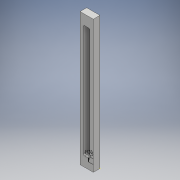
# Autodesk Inventor part: piças
Saved by Autodesk Inventor 2018 (Build 220112000, 112)
## iProperties
Created: 2018-03-15
Part Number: piças
Material: Genérico
Document SubType Name: Modeling
Designer: Georgines
Density: 1 g/cm^3
Appearance: Padrão
Author: Georgines
Autodesk Inventor part; units mm, degrees
ref_plane "YZ Plane" through (0, 0, 0) normal (1, 0, 0) x (0, 1, 0)
ref_plane "XZ Plane" through (0, 0, 0) normal (0, 1, 0) x (-1, 0, 0)
ref_plane "XY Plane" through (0, 0, 0) normal (0, 0, 1) x (1, 0, 0)
sketch "Esboço1" plane through (0, 0, 0) normal (0, 1, 0) x (-1, 0, 0)
  line L0 (-10, 100) -> (10, 100)
  line L1 (10, 100) -> (10, -100)
  line L2 (10, -100) -> (-10, -100)
  line L3 (-10, -100) -> (-10, 100)
  line L4 (-10, 100) -> (10, -100) construction
  line L5 (10, 100) -> (-10, -100) construction
  line L6 (-3, -85) -> (3, -85)
  line L7 (5, -83) -> (5, 83)
  line L8 (3, 85) -> (-3, 85)
  line L9 (-5, 83) -> (-5, -83)
  line L10 (-5, -85) -> (5, 85) construction
  line L11 (5, -85) -> (-5, 85) construction
  arc A0 (5, 83) -> (3, 85) centre (3, 83) ccw
  arc A1 (-3, 85) -> (-5, 83) centre (-3, 83) ccw
  arc A2 (3, -85) -> (5, -83) centre (3, -83) ccw
  arc A3 (-5, -83) -> (-3, -85) centre (-3, -83) ccw
  point P0 (0, 0)
  dimension "d0" = 20
  dimension "d1" = 200
  dimension "d2" = 10
  dimension "d3" = 170
  dimension "d6" = 2
  constraints: 24 end point, 8 point on circle, 8 point on line, 8 tangent, 4 centre point, 4 midpoint, 4 parallel, 3 equal radius, 2 horizontal, 2 perpendicular
  measures "d0" distance of L1.end L2.end
  measures "d1" distance of L0.end L1.end
  measures "d2" distance of L11.end L10.end
  measures "d3" distance of L10.end L11.start
  measures "d6" radius of A0
extrude "Extrusão1" add sketch "Esboço1" along normal blind 10
sketch "Esboço2" plane through (0, 10, 0) normal (0, 1, 0) x (1, 0, 0)
  line L0 (3, 85) -> (-3, 85) projected
  line L1 (0, 85) -> (0, 100) construction
  line L2 (10, 100) -> (-10, 100) projected
  line L3 (0, 85) -> (0, 92.5)
  point P0 (0, 0)
  point P1 (5, 85)
  point P2 (-5, 85)
  dimension "d7" = 15
  dimension "d8" = 7.5
  constraints: 4 end point, 3 midpoint
  measures "d7" distance of L1.start L1.end
  measures "d8" distance of L1.start L3.end
